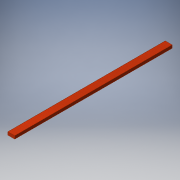
# Autodesk Inventor part: Lumber 2x4x80
Saved by Autodesk Inventor 2016 (Build 200138000, 138)
## iProperties
Created: 2015-05-30
Part Number: Lumber 2x4x80
Material: Wood (Oak)
Document SubType Name: Modeling
Designer: steele
Density: 0.76 g/cm^3
Appearance: White Oak - Natural Medium Gloss
Author: steele
Autodesk Inventor part; units mm, degrees
ref_plane "YZ Plane" through (0, 0, 0) normal (1, 0, 0) x (0, 1, 0)
ref_plane "XZ Plane" through (0, 0, 0) normal (0, 1, 0) x (-1, 0, 0)
ref_plane "XY Plane" through (0, 0, 0) normal (0, 0, 1) x (1, 0, 0)
sketch "Sketch1" plane through (0, 0, 0) normal (1, 0, 0) x (0, 1, 0)
  line L0 (-19.05, 1016) -> (-19.05, -1016)
  line L1 (-19.05, -1016) -> (19.05, -1016)
  line L2 (19.05, -1016) -> (19.05, 1016)
  line L3 (19.05, 1016) -> (-19.05, 1016)
  line L4 (-19.05, 1016) -> (19.05, -1016) construction
  line L5 (-19.05, -1016) -> (19.05, 1016) construction
  point P0 (0, 0)
  dimension "d0" = 38.1
  dimension "d1" = 2032
  constraints: 12 end point, 2 midpoint, 2 parallel, 1 perpendicular, 1 vertical
  measures "d0" distance of L0.end L1.end
  measures "d1" distance of L1.end L2.end
extrude "Extrusion1" add sketch "Sketch1" along normal blind 88.9
body "Solid1"
